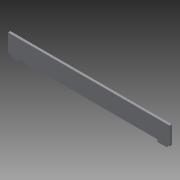
# Autodesk Inventor part: Side Wall 2
Saved by Autodesk Inventor 2013 (Build 170138000, 138)
## iProperties
Created: 2013-01-28
Part Number: Side Wall 2
Material: Generic
Document SubType Name: Modeling
Designer: Andrew Toennies
Density: 1 g/cm^3
Author: Andrew Toennies
Autodesk Inventor part; units mm, degrees
ref_plane "YZ Plane" through (0, 0, 0) normal (1, 0, 0) x (0, 1, 0)
ref_plane "XZ Plane" through (0, 0, 0) normal (0, 1, 0) x (-1, 0, 0)
ref_plane "XY Plane" through (0, 0, 0) normal (0, 0, 1) x (1, 0, 0)
sketch "Sketch1" plane through (0, 0, 0) normal (0, 0, 1) x (1, 0, 0)
  line L0 (0, 0) -> (3.175, 0)
  line L1 (3.175, 0) -> (3.175, -3.175)
  line L2 (3.175, -3.175) -> (15.875, -3.175)
  line L3 (15.875, -3.175) -> (15.875, 0)
  line L4 (0, 0) -> (0, 25.4)
  line L5 (307.975, 25.4) -> (307.975, 0)
  line L6 (307.975, 0) -> (15.875, 0)
  line L7 (0, 25.4) -> (-11.8442, 50.8)
  line L8 (307.975, 25.4) -> (263.9809, 50.8)
  line L9 (-11.8442, 50.8) -> (263.9809, 50.8)
  dimension "d0" = 3.175
  dimension "d1" = 3.175
  dimension "d2" = 12.7
  dimension "d3" = 25.4
  dimension "d4" = 307.975
  dimension "d12" = 25.4
  dimension "d13" = 25
  dimension "d14" = 60
  constraints: 20 end point, 4 parallel, 2 horizontal, 2 perpendicular, 1 vertical
  measures "d0" distance of L0.start L0.end
  measures "d1" distance of L0.end L1.end
  measures "d2" distance of L1.end L2.end
  measures "d3" distance of L0.start L4.end
  measures "d4" distance of L4.end L5.start
  measures "d12" distance from line of L9 L4.end
  measures "d13" angle of L7 L4
  measures "d14" angle of L8 L5
extrude "Extrusion1" add sketch "Sketch1" along normal blind 3.175
sketch "Sketch2" plane through (0, 0, 3.175) normal (0, 0, 1) x (1, 0, 0)
  line L0 (286.9872, 0) -> (299.6872, 0) projected
  line L1 (286.9872, -3.175) -> (286.9872, 0) projected
  line L2 (299.6872, -3.175) -> (286.9872, -3.175) projected
  line L3 (299.6872, 0) -> (299.6872, -3.175) projected
extrude "Extrusion2" add sketch "Sketch2" against normal blind 3.175
body "Solid1"
